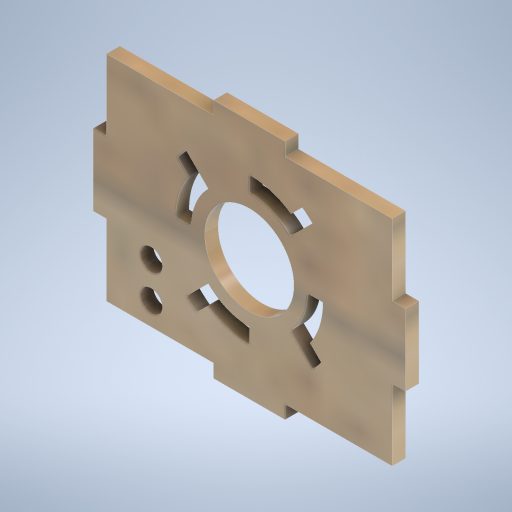
# Autodesk Inventor part: back plate
Saved by Autodesk Inventor 2023 (Build 270158000, 158)
## iProperties
Created: 2023-06-06
Part Number: back plate
Material: Hardboard
Document SubType Name: Sheet Metal
Designer: Ronan
Density: 0.799949 g/cm^3
Sheet Metal Rule: Default_mm
Appearance: Natural Maple - Glossy Dark Tint(1)
Author: Ronan
Autodesk Inventor part; units mm, degrees
ref_plane "YZ Plane" through (0, 0, 0) normal (1, 0, 0) x (0, 1, 0)
ref_plane "XZ Plane" through (0, 0, 0) normal (0, 1, 0) x (-1, 0, 0)
ref_plane "XY Plane" through (0, 0, 0) normal (0, 0, 1) x (1, 0, 0)
sketch "Sketch1" plane through (0, 0, 0) normal (0, 0, 1) x (1, 0, 0)
  line L0 (-24, 48) -> (-24, 51)
  line L1 (-24, 51) -> (-40, 51)
  line L2 (-40, 51) -> (-40, 48)
  line L3 (0, 32) -> (3, 32)
  line L4 (3, 32) -> (3, 16)
  line L5 (3, 16) -> (0, 16)
  line L6 (-40, 0) -> (-40, -3)
  line L7 (-40, -3) -> (-24, -3)
  line L8 (-24, -3) -> (-24, 0)
  line L9 (-64, 16) -> (-67, 16)
  line L10 (-67, 16) -> (-67, 32)
  line L11 (-67, 32) -> (-64, 32)
  line L12 (-64, 48) -> (-40, 48)
  line L13 (-24, 48) -> (0, 48)
  line L14 (-64, 0) -> (-64, 16)
  line L15 (-64, 32) -> (-64, 48)
  line L16 (0, 0) -> (-24, 0)
  line L17 (-40, 0) -> (-64, 0)
  line L18 (0, 48) -> (0, 32)
  line L19 (0, 16) -> (0, 0)
  point P0 (0, 0)
  dimension "d3" = 16
  dimension "d4" = 16
  dimension "d8" = 64
  dimension "d9" = 48
  dimension "d10" = 3
  dimension "d11" = 3
  dimension "d12" = 24
  dimension "d13" = 24
  dimension "d14" = 16
  dimension "d15" = 3
  measures "d3" distance of L0.end L1.end
  measures "d4" distance of L3.end L4.end
  measures "d8" distance between parallel lines of L18 L15
  measures "d9" distance between parallel lines of L17 L12
  measures "d10" distance of L10.end L11.end
  measures "d11" distance of L6.start L6.end
  measures "d12" distance of L0.start L13.end
  measures "d13" distance of L12.start L2.end
  measures "d14" distance of L6.end L7.end
  measures "d15" distance of L1.end L2.end
extrude "Plate1" add sketch "Sketch1" along normal blind 3
sketch "Sketch2" plane through (0, 0, 3) normal (0, 0, 1) x (1, 0, 0)
  circle A0 centre (-32, 24) radius 10
  line L0 (-67, 32) -> (-67, 16) projected
  line L1 (-40, 51) -> (-24, 51) projected
  line L2 (0, 0) -> (0, 16) projected
  circle A1 centre (-32, 24) radius 16.5
  circle A2 centre (-32, 24) radius 20
  line L3 (0, 0) -> (-24, 0) projected
  line L4 (-64, 32) -> (-64, 48) projected
  line L5 (0, 48) -> (0, 32) projected
  line L6 (-64, 48) -> (-40, 48) projected
  line L7 (-64, 0) -> (-40, 0) projected
  line L8 (-52, 24) -> (-12, 24)
  line L9 (-32, 44) -> (-32, 4)
  line L10 (-17.8579, 38.1421) -> (-46.1421, 9.8579)
  line L11 (-17.8579, 9.8579) -> (-46.1421, 38.1421)
  line L12 (-22.6485, 37.5941) -> (-20.1392, 40.1035)
  line L13 (-18.4059, 14.6485) -> (-15.8965, 12.1392)
  line L14 (-41.3515, 10.4059) -> (-43.8608, 7.8965)
  line L15 (-45.5941, 33.3515) -> (-48.1035, 35.8608)
  circle A3 centre (-32, 24) radius 13
  circle A4 centre (-54, 5) radius 2.5
  circle A5 centre (-54, 13) radius 2.5
  line L16 (-64, 0) -> (-64, 16) projected
  point P0 (-32, 24)
  point P1 (-17.1512, 13.3939)
  point P2 (-32, 37)
  point P3 (-22.8076, 33.1924)
  point P4 (-32, 40.5)
  point P5 (-19, 24)
  point P6 (-22.8076, 14.8076)
  point P7 (-48.5, 24)
  point P8 (-32, 11)
  point P9 (-41.1924, 14.8076)
  point P10 (-32, 7.5)
  point P11 (-15.5, 24)
  point P12 (-45, 24)
  point P13 (-41.1924, 33.1924)
  point P14 (-43.6673, 35.6673)
  point P15 (-32, 24)
  point P16 (-20.3327, 12.3327)
  dimension "d17" = 20
  dimension "d21" = 3.5
  dimension "d24" = 24
  dimension "d25" = 32
  dimension "d26" = 45
  dimension "d27" = 3
  dimension "d28" = 3
  dimension "d29" = 3
  dimension "d30" = 3
  dimension "d31" = 3
  dimension "d34" = 5
  dimension "d35" = 5
  dimension "d36" = 5
  dimension "d37" = 10
  dimension "d38" = 8
  dimension "d39" = 3.5
  constraints: 16 end point, 8 midpoint, 5 centre point, 4 parallel, 4 point on circle, 3 coincident, 2 perpendicular, 1 vertical, 1 vertical alignment, 14 other
  measures "d17" diameter of A0
  measures "d24" vertical distance of L2.start A0.centre
  measures "d25" horizontal distance of L2.start A0.centre
  measures "d26" angle of L10 L9
  measures "d27" distance between parallel lines of L10 L12
  measures "d28" distance between parallel lines of L11 L15
  measures "d29" distance between parallel lines of L10 L14
  measures "d30" distance from line of L11 point (-17.151, 13.394)
  measures "d31" radial gap between concentric circles of A0 A3
  measures "d34" diameter of A4
  measures "d35" diameter of A5
  measures "d36" distance from line of L7 A4.centre
  measures "d37" distance from line of L16 A4.centre
  measures "d38" distance of A5.centre A4.centre
  measures "d39" radial gap between concentric circles of A3 A1
extrude "Extrusion1" cut sketch "Sketch2" against normal through all contours L8 L10 A0 | A0 L11 L8 | L10 L9 A0 | A0 L9 L11 | L8 A1 L11 A3 | L10 A0 L8 | L11 A0 L9 | L9 A0 L10 | L8 A0 L11 | A3 L9 A1 L10 | A1 L12 A2 L10 | L9 A1 L10 A3 | A1 L13 A2 L11 | L8 A1 L11 A3 | A1 L14 A2 L10 | A1 L15 A2 L11 | A4 | A5
equation "\"d16\" = Thickness"
equation "\"BendRadius\" = Thickness"
equation "\"BendReliefWidth\" = Thickness"
equation "\"BendReliefDepth\" = 0.5 * Thickness"
equation "\"CornerReliefSize\" = 4 * Thickness"
equation "\"MinimumRemnant\" = 2 * Thickness"
equation "\"TransitionRadius\" = BendRadius"
equation "\"JacobiRadiusSize\" = BendRadius"
equation "\"GapSize\" = Thickness"
equation "\"Thickness\" = 3"
body "Solid1"
